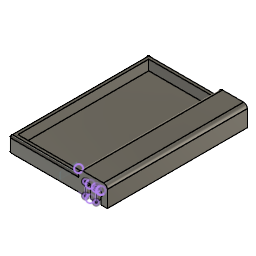
schrankAblage (Autodesk Fusion 360 design; units mm, degrees)
part number: 2025-06-24-21-58-04-379
Autodesk Fusion 360 part; units mm, degrees
note: some values were not read from the file. Chosen so that the rebuilt part matches the saved one: which face or edge a step refers to; a direction; which sketch regions a step uses.
sketch "Skizze1" plane through (0, 0, 0) normal (0, 1, 0) x (1, 0, 0)
  line L0 (4.31, -11.7) -> (-0.69, -11.7)
  line L1 (-8, -17.7) -> (-8, 1.8288)
  line L2 (10.8, -11.7) -> (15.8, -11.7)
  line L3 (4.31, -11.7) -> (4.31, 1.8288)
  line L4 (15.8, -11.7) -> (15.8, 1.8288)
  line L5 (15.8, 1.8288) -> (22.6, 1.8288)
  line L6 (22.6, 1.8288) -> (22.6, -19.9712)
  line L7 (22.6, -19.9712) -> (-8, -19.9712)
  line L8 (-8, -19.9712) -> (-8, -17.7)
  line L9 (10.8, -11.7) -> (10.8, 1.8288)
  line L10 (10.8, 1.8288) -> (4.31, 1.8288)
  line L11 (-0.69, -11.7) -> (-0.69, 1.8288)
  line L12 (-0.69, 1.8288) -> (-8, 1.8288)
  dimension "d26" = 5
  dimension "d33" = 5
  dimension "d49" = 21.8
  constraint perpendicular L0 L3
  constraint perpendicular L2 L4
  constraint perpendicular L5 L6
  constraint perpendicular L1 L7
  constraint perpendicular L7 L8
  constraint vertical L1
  constraint coincident L1 L12.end
  constraint perpendicular L2 L9
  constraint perpendicular L3 L10
  constraint perpendicular L0 L11
  constraint perpendicular L1 L12
  measures "d26" distance of L0.start L0.end
  measures "d33" distance of L2.start L2.end
  measures "d49" distance of L5.end L6.end
extrude "Extrusion1" add sketch "Skizze1" along normal blind 150
sketch "Skizze2" plane through (0, 150, 0) normal (0, 1, 0) x (-1, 0, 0)
  line L0 (-4.31, 11.7) -> (0.69, 11.7)
  line L1 (8, -1.8288) -> (8, 19.9712)
  line L2 (21, 3.5) -> (24.5, 7)
  line L3 (24.5, 7) -> (21, 7)
  line L4 (-15.8, 11.7) -> (-10.8, 11.7)
  line L5 (-22.6, -1.8288) -> (-15.8, -1.8288)
  line L6 (-15.8, -1.8288) -> (-15.8, 11.7)
  line L7 (-4.31, -1.8288) -> (-4.31, 11.7)
  line L8 (8, 19.9712) -> (-22.6, 19.9712)
  line L9 (-22.6, 19.9712) -> (-22.6, -1.8288)
  line L10 (0.69, 11.7) -> (0.69, -1.8288)
  line L11 (0.69, -1.8288) -> (8, -1.8288)
  line L12 (-10.8, 11.7) -> (-10.8, -1.8288)
  line L13 (-10.8, -1.8288) -> (-4.31, -1.8288)
extrude "Extrusion2" cut sketch "Skizze2" along normal blind 46
sketch "Skizze3" plane through (-28, 0, 0) normal (-1, 0, 0) x (0, -1, 0)
  line L0 (0, 0) -> (0, 7)
  line L1 (0, 7) -> (-18, 7)
  line L2 (-18, 7) -> (-18, 0)
  line L3 (-18, 0) -> (0, 0)
  dimension "d15" = 18
  measures "d15" distance of L0.end L1.end
sketch "Skizze4" plane through (0, 0, 0) normal (0, -1, 0) x (1, 0, 0)
  line L0 (-8, 19.9712) -> (-8, -1.8288)
  line L1 (-0.69, 11.7) -> (4.31, 11.7)
  line L2 (10.8, 11.7) -> (15.8, 11.7)
  line L3 (4.31, -1.8288) -> (10.8, -1.8288)
  line L4 (10.8, -1.8288) -> (10.8, 11.7)
  line L5 (-8, -1.8288) -> (-0.69, -1.8288)
  line L6 (-0.69, -1.8288) -> (-0.69, 11.7)
sketch "Skizze5" plane through (0, 0, 0) normal (0, -1, 0) x (1, 0, 0)
sketch "Skizze6" plane through (0, 0, 0) normal (0, -1, 0) x (1, 0, 0)
sketch "Skizze7" plane through (0, 0, 0) normal (0, -1, 0) x (1, 0, 0)
  line L0 (10.8, 11.7) -> (15.8, 11.7)
  dimension "d38" = 5
  measures "d38" distance of L0.start L0.end
sketch "Skizze8" plane through (0, 0, 0) normal (0, -1, 0) x (1, 0, 0)
  line L0 (-0.19, 11.7) -> (4.31, 11.7)
  line L1 (10.8, 11.7) -> (15.8, 11.7)
  line L2 (4.31, -1.8288) -> (11.3, -1.8288)
  line L3 (7.805, -1.8288) -> (7.805, 17.6356)
  circle A0 centre (1.4444, 8.4164) radius 3.15
  circle A1 centre (14.1656, 8.4164) radius 3.15
  dimension "d43" = 4.5
  dimension "d44" = 5
  dimension "d45" = 6.99
  dimension "d46" = 6.3
  constraint midpoint L2 L3.start
  constraint perpendicular L2 L3
  constraint symmetric L3 A0 A1
  measures "d43" distance of L0.start L0.end
  measures "d44" distance of L1.start L1.end
  measures "d45" distance of L2.start L2.end
  measures "d46" diameter of A0
extrude "Extrusion3" cut sketch "Skizze8" against normal blind 180
fillet "Abrundung8" radius 4 2 edges at (-8, 75, 19.9712) (22.6, 75, 19.9712)
sketch "Skizze9" plane through (-8, 0, 0) normal (-1, 0, 0) x (0, -1, 0)
  line L0 (0, 15.9712) -> (-150, 15.9712)
  line L1 (-150, 15.9712) -> (-150, -1.8288)
  line L2 (0, -1.8288) -> (0, 15.9712)
  line L3 (0, -1.8288) -> (-150, -1.8288)
  line L4 (-150, -1.8288) -> (-150, 14)
  line L5 (-150, 14) -> (0, 14)
  line L6 (0, 14) -> (0, -1.8288)
  line L7 (-150, -1.8288) -> (0, -1.8288)
  constraint horizontal L3
  constraint vertical L4
  constraint horizontal L5
  constraint vertical L6
  constraint coincident L1 L4.end
  constraint coincident L2.start L3.start
extrude "Extrusion4" add sketch "Skizze9" along normal blind 75 contours L1 L2 L3 L4 L5 L6 L7
shell "Schale1" thickness 5 removed faces 1 at (-33, 100, 14)
fillet "Abrundung9" radius 2 2 edges at (-83, 0, 6.0856) (-83, 150, 6.0856)
fillet "Abrundung10" radius 2 5 edges at (-44.5, 0, 14) (-82.4142, 0.5858, 14) (-83, 75, 14) (-82.4142, 149.4142, 14) (-44.5, 150, 14)
